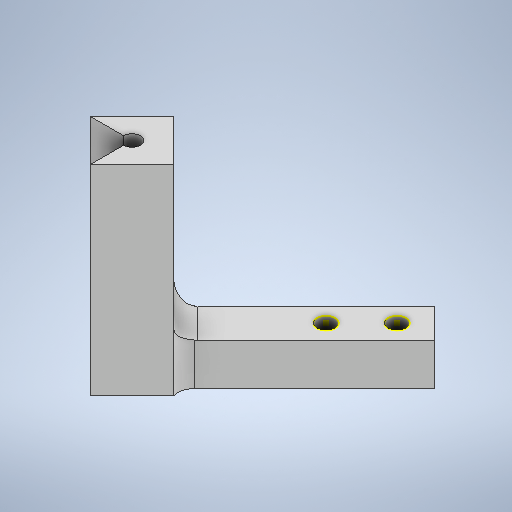
# Autodesk Inventor part: ALUMFINGER
Saved by Autodesk Inventor 2025.1 (Build 291241000, 241)
## iProperties
Created: 2025-02-25
Part Number: ALUMFINGER
Material: Generic
Document SubType Name: Modeling
Designer: m_kni
Density: 1 g/cm^3
Appearance: Default
Author: m_kni
## iProperties of the stored document ALUMFINGER_3DPrint.ipt
Created: 2025-03-03
Part Number: ALUMFINGER_3DPrint
Material: Generic
Document SubType Name: Modeling
Designer: m_kni
Density: 1 g/cm^3
Appearance: Default
Author: m_kni
Autodesk Inventor part; units mm, degrees
ref_plane "YZ Plane" through (0, 0, 0) normal (1, 0, 0) x (0, 1, 0)
ref_plane "XZ Plane" through (0, 0, 0) normal (0, 1, 0) x (-1, 0, 0)
ref_plane "XY Plane" through (0, 0, 0) normal (0, 0, 1) x (1, 0, 0)
sketch "Sketch1" plane through (0, 0, 0) normal (0, 1, 0) x (-1, 0, 0)
  arc A0 (-0.158902, 2.527129) -> (-1.647898, 1.801809) centre (0.148153, 0.005757) ccw
  arc A1 (-0.158902, 2.527129) -> (-1.647898, 1.801809) centre (0.148153, 0.005757) ccw
  arc A2 (1.944204, -1.790294) -> (2.669525, -0.301298) centre (0.148153, 0.005757) ccw
  arc A3 (1.944204, -1.790294) -> (2.669525, -0.301298) centre (0.148153, 0.005757) ccw
  arc A4 (0.148153, 2.545757) -> (-1.647898, 1.801809) centre (0.148153, 0.005757) ccw
  line L0 (0.148153, 5.005757) -> (0.148153, 2.545757)
  line L1 (0.148153, 0.005757) -> (2.688153, 0.005757)
  line L2 (-1.647898, 1.801809) -> (-4.147898, -0.698191)
  arc A5 (1.944204, -1.790294) -> (2.688153, 0.005757) centre (0.148153, 0.005757) ccw
  line L3 (-4.147898, -0.698191) -> (-4.851847, 0.005757)
  arc A6 (0.148153, 2.545757) -> (-1.647898, 1.801809) centre (0.148153, 0.005757) ccw
  arc A7 (0.148153, 2.545757) -> (-1.647898, 1.801809) centre (0.148153, 0.005757) ccw
  arc A8 (-0.158902, 2.527129) -> (-1.647898, 1.801809) centre (0.148153, 0.005757) ccw
  arc A9 (-0.158902, 2.527129) -> (-1.647898, 1.801809) centre (0.148153, 0.005757) ccw
  line L4 (-4.851847, 0.005757) -> (0.148153, 5.005757)
  line L5 (-4.851847, 0.005757) -> (0.148153, 5.005757)
  line L6 (0.148153, 5.005757) -> (0.148153, 2.545757)
  arc A10 (0.148153, 2.545757) -> (-1.647898, 1.801809) centre (0.148153, 0.005757) ccw
  line L7 (-1.647898, 1.801809) -> (-4.147898, -0.698191)
  line L8 (-4.147898, -0.698191) -> (-4.851847, 0.005757)
  arc A11 (1.944204, -1.790294) -> (2.688153, 0.005757) centre (0.148153, 0.005757) ccw
  arc A12 (1.944204, -1.790294) -> (2.669525, -0.301298) centre (0.148153, 0.005757) ccw
  arc A13 (1.944204, -1.790294) -> (2.669525, -0.301298) centre (0.148153, 0.005757) ccw
  arc A14 (1.944204, -1.790294) -> (2.688153, 0.005757) centre (0.148153, 0.005757) ccw
  line L9 (-4.147898, -0.698191) -> (-0.555796, -4.290294)
  line L10 (0.148153, 1.005757) -> (0.148153, 0.005757)
  line L11 (0.148153, 1.005757) -> (0.148153, 0.005757)
  line L12 (0.148153, 2.545757) -> (0.148153, 0.005757)
  line L13 (0.148153, 5.005757) -> (0.148153, 2.545757)
  line L14 (0.148153, 5.005757) -> (0.148153, 1.005757)
  line L15 (0.148153, 0.005757) -> (1.148153, 0.005757)
  line L16 (1.148153, 0.005757) -> (5.148153, 0.005757)
  line L17 (2.688153, 0.005757) -> (5.148153, 0.005757)
  line L18 (0.148153, 0.005757) -> (2.688153, 0.005757)
  line L19 (5.148153, 0.005757) -> (0.148153, -4.994243)
  line L20 (0.148153, -4.994243) -> (5.148153, 0.005757)
  line L21 (-4.147898, -0.698191) -> (-4.851847, 0.005757)
  line L22 (-4.147898, -0.698191) -> (-0.555796, -4.290294)
  line L23 (0.148153, -4.994243) -> (-0.555796, -4.290294)
  line L24 (-4.851847, 0.005757) -> (0.148153, -4.994243)
  line L25 (-4.851847, 0.005757) -> (0.148153, -4.994243)
  line L26 (0.148153, 5.005757) -> (-4.851847, 0.005757)
  line L27 (-4.851847, 0.005757) -> (0.148153, 5.005757)
  line L28 (0.148153, 5.005757) -> (-4.851847, 0.005757)
  line L29 (0.148153, -4.994243) -> (-0.555796, -4.290294)
  arc A15 (1.944204, -1.790294) -> (2.688153, 0.005757) centre (0.148153, 0.005757) ccw
  line L30 (-0.555796, -4.290294) -> (1.944204, -1.790294)
  line L31 (2.688153, 0.005757) -> (5.148153, 0.005757)
  line L32 (5.148153, 0.005757) -> (0.148153, -4.994243)
  line L33 (0.148153, -4.994243) -> (-0.555796, -4.290294)
  line L34 (-0.555796, -4.290294) -> (1.944204, -1.790294)
  arc A16 (1.944204, -1.790294) -> (2.688153, 0.005757) centre (0.148153, 0.005757) ccw
  line L35 (2.688153, 0.005757) -> (5.148153, 0.005757)
  line L36 (5.148153, 0.005757) -> (0.148153, -4.994243)
  arc A17 (0.148153, 2.545757) -> (-1.647898, 1.801809) centre (0.148153, 0.005757) ccw
  circle A18 centre (-2.355005, -2.497401) radius 1.5
  circle A19 centre (-2.355005, -2.497401) radius 1.5
  circle A20 centre (-2.355005, -2.497401) radius 1.5
  circle A21 centre (-2.355005, -2.497401) radius 1.5
  circle A22 centre (-2.355005, -2.497401) radius 1.5
  line L37 (0.148153, 5.005757) -> (0.148153, 1.005757)
  arc A23 (0.148153, 1.005757) -> (1.148153, 0.005757) centre (0.148153, 0.005757) ccw
  line L38 (0.148153, -4.994243) -> (5.148153, 0.005757)
  line L39 (1.148153, 0.005757) -> (5.148153, 0.005757)
  line L40 (0.148153, 0.005757) -> (1.148153, 0.005757)
  arc A24 (0.148153, 1.005757) -> (1.148153, 0.005757) centre (0.148153, 0.005757) ccw
  line L41 (0.148153, 0.005757) -> (1.148153, 0.005757)
  line L42 (0.148153, 1.005757) -> (0.148153, 0.005757)
  arc A25 (0.148153, 1.005757) -> (1.148153, 0.005757) centre (0.148153, 0.005757) ccw
  arc A26 (0.148153, 1.005757) -> (1.148153, 0.005757) centre (0.148153, 0.005757) ccw
  arc A27 (0.148153, 1.005757) -> (1.148153, 0.005757) centre (0.148153, 0.005757) ccw
  line L43 (0.148153, 5.005757) -> (-4.851847, 0.005757)
  line L44 (-4.851847, 0.005757) -> (0.148153, -4.994243)
  line L45 (0.148153, -4.994243) -> (5.148153, 0.005757)
  line L46 (1.148153, 0.005757) -> (5.148153, 0.005757)
  arc A28 (0.148153, 1.005757) -> (1.148153, 0.005757) centre (0.148153, 0.005757) ccw
  line L47 (0.148153, 5.005757) -> (0.148153, 1.005757)
  line L48 (0.148153, 2.545757) -> (0.148153, 0.005757)
  arc A29 (-1.647898, 1.801809) -> (1.944204, -1.790294) centre (0.148153, 0.005757) ccw
  circle A30 centre (0.148153, 0.005757) radius 2.54
  line L49 (0.148153, -3.586345) -> (-3.443949, 0.005757)
  line L50 (-1.647898, -1.790294) -> (-2.355005, -2.497401)
  circle A31 centre (-2.355005, -2.497401) radius 2.54
  point P0 (0, 0)
  point P1 (1.148153, 0.005757)
  constraints: 86 end point, 44 point on circle, 28 centre point, 38 other
extrude "Extrusion1" add sketch "Sketch1" along normal blind 23.9 contours A4 L12 A23 A31 A29 A0 | A0 L2 L3 L4 L0 A4 | A29 A31 L49 L2 | L49 A31 L2 | A31 A29 A18 | A29 A18 L49 A31 | A5 A2 A29 A31 A23 L1 | L16 L19 L23 L30 A2 A5 | A31 L49 A18 L9 | A29 L49 A18 | A18 A29 | A18 L49 L50 L9 | A31 L49 L30 | L9 A18 L49 A31 | A29 A31 L49 A18 | A18 L49 A29 | L49 A18 L9 L50 | L30 L49 A31 A29
sketch "Sketch2" plane through (0, 0, 0) normal (0, -1, 0) x (1, 0, 0)
  line L0 (4.851847, 0.005757) -> (-0.148153, -4.994243)
  line L1 (2.351847, -2.494243) -> (17.908196, -18.050592)
  circle A0 centre (11.448069, -11.590464) radius 1.075
  circle A1 centre (15.690709, -15.833105) radius 1.075
  line L2 (-0.148153, 1.005757) -> (-0.148153, 5.005757)
  line L3 (-0.148153, 5.005757) -> (4.851847, 0.005757)
  line L4 (-0.148153, 5.005757) -> (4.851847, 0.005757)
  line L5 (-0.148153, -4.994243) -> (-5.148153, 0.005757)
  line L6 (-5.148153, 0.005757) -> (-0.148153, -4.994243)
  line L7 (2.351847, -2.494243) -> (4.119614, -0.726476)
  line L8 (4.119614, -0.726476) -> (0.58408, -4.26201)
  line L9 (0.58408, -4.26201) -> (16.044263, -19.722192)
  line L10 (4.119614, -0.726476) -> (19.579797, -16.186658)
  line L11 (17.908196, -18.050592) -> (17.81203, -18.146758)
  line L12 (17.81203, -18.146758) -> (16.140429, -19.818359)
  line L13 (16.140429, -19.818359) -> (16.044263, -19.722192)
  line L14 (17.908196, -18.050592) -> (19.675963, -16.282825)
  line L15 (19.675963, -16.282825) -> (19.579797, -16.186658)
  point P0 (0, 0)
  dimension "d2" = 22
  dimension "d5" = 2.15
  dimension "d6" = 2.15
  dimension "d7" = 2.5
  dimension "d8" = 5
  constraints: 24 end point, 8 point on line, 3 perpendicular, 2 centre point, 2 collinear, 1 midpoint
  measures "d2" distance of L1.start L1.end
  measures "d5" diameter of A0
  measures "d6" diameter of A1
  measures "d7" distance of L1.start L7.end
  measures "d8" distance of L7.end L8.end
extrude "Extrusion2" add sketch "Sketch2" against normal blind 5 contours L10 L15 L14 L1 A1 A0 L0 | L1 A0 A1 L11 L12 L13 L9 L0
fillet "Fillet1" radius 2 2 edges at (4.1196, 2.5, -0.7265) (0.5841, 2.5, -4.262)
fillet "Fillet2" radius 2 1 edges at (2.3518, 5, -2.4942)
sketch "Sketch3" plane through (0, 5, 0) normal (0, 1, 0) x (1, 0, 0)
  circle A0 centre (11.448069, 11.590464) radius 1.075
  circle A1 centre (15.690709, 15.833105) radius 1.075
  point P0 (0, 0)
body "Solid1"
